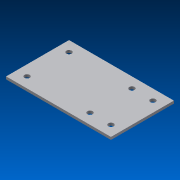
# Autodesk Inventor part: MountSwitchBar
Saved by Autodesk Inventor 2013 (Build 170138000, 138)
## iProperties
Created: 2013-07-20
Part Number: MountSwitchBar
Material: Aluminum 6061
Document SubType Name: Modeling
Designer: robotics
Density: 1 g/cm^3
Author: robotics
Autodesk Inventor part; units mm, degrees
ref_plane "YZ Plane" through (0, 0, 0) normal (1, 0, 0) x (0, 1, 0)
ref_plane "XZ Plane" through (0, 0, 0) normal (0, 1, 0) x (-1, 0, 0)
ref_plane "XY Plane" through (0, 0, 0) normal (0, 0, 1) x (1, 0, 0)
sketch "Sketch1" plane through (0, 0, 0) normal (0, 1, 0) x (-1, 0, 0)
  line L0 (0, 0) -> (127, 0)
  line L1 (127, 0) -> (127, 76.2)
  line L2 (127, 76.2) -> (0, 76.2)
  line L3 (0, 76.2) -> (0, 0)
  dimension "d0" = 127
  dimension "d2" = 76.2
  constraints: 8 end point, 2 parallel, 1 horizontal, 1 perpendicular
  measures "d0" distance of L1.end L2.end
  measures "d2" distance of L2.end L0.start
extrude "Extrusion1" add sketch "Sketch1" along normal blind 3.175
sketch "Sketch2" plane through (0, 0, 0) normal (0, -1, 0) x (1, 0, 0)
  line L0 (0, 0) -> (-127, 0) projected
  line L1 (0, 76.2) -> (0, 0) projected
  line L2 (-127, 76.2) -> (0, 76.2) projected
  line L3 (-127, 0) -> (-127, 76.2) projected
  point P0 (-114.3, 63.5)
  point P1 (-12.7, 63.5)
  point P2 (-12.7, 12.7)
  point P3 (-114.3, 12.7)
  dimension "d5" = 12.7
  dimension "d6" = 12.7
  dimension "d7" = 12.7
  dimension "d8" = 12.7
  dimension "d9" = 12.7
  dimension "d10" = 12.7
  dimension "d11" = 12.7
  dimension "d12" = 12.7
  measures "d5" distance from line of L0 point (-114.3, 12.7)
  measures "d6" distance from line of L3 point (-114.3, 12.7)
  measures "d7" distance from line of L3 point (-114.3, 63.5)
  measures "d8" distance from line of point (-114.3, 63.5) L2
  measures "d9" distance from line of L1 point (-12.7, 12.7)
  measures "d10" distance from line of L0 point (-12.7, 12.7)
  measures "d11" distance from line of point (-12.7, 63.5) L2
  measures "d12" distance from line of L1 point (-12.7, 63.5)
hole "Hole1" at (-114.3, 0, 63.5) at (-12.7, 0, 63.5) at (-12.7, 0, 12.7) at (-114.3, 0, 12.7) direction (0, 1, 0) diameter 6.35 end through all
sketch "Sketch3" plane through (0, 3.175, 0) normal (0, 1, 0) x (1, 0, 0)
  line L0 (-127, -76.2) -> (0, -76.2) projected
  line L1 (0, -76.2) -> (0, 0) projected
  line L2 (0, 0) -> (-127, 0) projected
  point P0 (-38.1, -63.5)
  point P1 (-38.1, -12.7)
  dimension "d20" = 12.7
  dimension "d21" = 38.1
  dimension "d29" = 12.7
  dimension "d30" = 38.1
  measures "d20" distance from line of L0 point (-38.1, -63.5)
  measures "d21" distance from line of L1 point (-38.1, -63.5)
  measures "d29" distance from line of point (-38.1, -12.7) L2
  measures "d30" distance from line of L1 point (-38.1, -12.7)
hole "Hole2" at (-38.1, 3.175, 63.5) at (-38.1, 3.175, 12.7) direction (0, -1, 0) diameter 6.35 end through all
body "Solid1"
